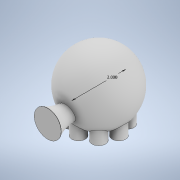
# Autodesk Inventor part: Head
Saved by Autodesk Inventor 2021 (Build 250183000, 183)
## iProperties
Created: 2020-07-13
Part Number: Head
Material: Generic
Document SubType Name: Modeling
Designer: saipr
Density: 1 g/cm^3
Appearance: Default
Author: saipr
Autodesk Inventor part; units mm, degrees
ref_plane "YZ Plane" through (0, 0, 0) normal (1, 0, 0) x (0, 1, 0)
ref_plane "XZ Plane" through (0, 0, 0) normal (0, 1, 0) x (-1, 0, 0)
ref_plane "XY Plane" through (0, 0, 0) normal (0, 0, 1) x (1, 0, 0)
sketch "Sketch1" plane through (0, 0, 0) normal (0, 0, 1) x (1, 0, 0)
  circle A0 centre (0, 0) radius 31.75
  line L0 (0, 0) -> (0, -7.62)
  circle A1 centre (0, -7.62) radius 7.62
  line L1 (0, 31.75) -> (0, -31.75)
  line L2 (25.4, -19.05) -> (12.7, -19.05)
  line L3 (12.7, -19.05) -> (12.7, -31.75)
  line L4 (25.4, -31.75) -> (25.4, -19.05)
  line L5 (19.05, -31.75) -> (19.05, -30.226)
  arc A2 (21.8353, -31.75) -> (16.2647, -31.75) centre (19.05, -30.226) ccw
  line L6 (12.7, -31.75) -> (16.2647, -31.75)
  line L7 (21.8353, -31.75) -> (25.4, -31.75)
  line L8 (19.05, -30.226) -> (19.05, -19.05)
  point P0 (19.05, -25.4)
  point P1 (19.05, -27.051)
  dimension "d0" = 63.5
  dimension "d1" = 7.62
  dimension "d12" = 12.7
  dimension "d13" = 12.7
  dimension "d14" = 1.524
  dimension "d15" = 6.35
  constraints: 18 end point, 5 point on circle, 3 coincident, 3 parallel, 3 vertical, 2 centre point, 2 tangent, 1 horizontal, 1 midpoint, 1 perpendicular, 1 vertical alignment, 2 other
  measures "d0" diameter of A0
  measures "d1" distance of L0.start L0.end
  measures "d12" distance of L4.start L3.end
  measures "d13" distance of L4.start L2.start
  measures "d14" distance of L5.start L5.end
  measures "d15" diameter of A2
sketch "Sketch2" plane through (0, 0, 0) normal (0, 1, 0) x (-1, 0, 0)
  circle A0 centre (0, 0) radius 25.4
  dimension "d2" = 50.8
  constraints: 1 centre point, 1 coincident
  measures "d2" diameter of A0
extrude "Extrusion1" add sketch "Sketch2" along normal mid plane 12.7
revolve "Revolution1" add sketch "Sketch1" angle 360 about axis through (0, 31.75, 0) along (0, -1, 0) picked at (3.5695, -11.1895) contours A0 L2 L3 L1 A1 | A0 L8 L2 | A1 L1 L0 | A0 L3 L2 L8
extrude "Extrusion2" add sketch "Sketch1" along normal blind 48.26 contours A1 L1 L0 | L0 L1 A1
sketch "Sketch3" plane through (0, -7.62, 48.26) normal (0, 0, 1) x (1, 0, 0)
  circle A0 centre (0, 0) radius 12.7
  point P0 (0, 7.62)
  dimension "d8" = 25.4
  constraints: 1 centre point
  measures "d8" diameter of A0
extrude "Extrusion3" add sketch "Sketch3" against normal blind 0.254
fillet "Fillet1" radius 40.64 1 edges at (-7.62, -7.62, 48.006)
revolve "Revolution2" add sketch "Sketch1" angle 360 about axis through (19.05, -30.226, 0) along (0, 1, 0) contours L4 L7 A2 L8 A0
pattern_circular "Circular Pattern1" count 8 over 360 about axis through (0, 0, 0) along (0, 1, 0) of "Revolution2"
body "Solid1"
